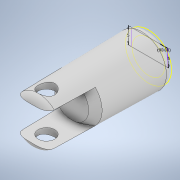
# Autodesk Inventor part: bicep
Saved by Autodesk Inventor 2021 (Build 250183000, 183)
## iProperties
Created: 2021-06-26
Part Number: bicep
Material: Generic
Document SubType Name: Modeling
Designer: TARUN
Density: 1 g/cm^3
Appearance: Default
Author: TARUN
Autodesk Inventor part; units mm, degrees
ref_plane "YZ Plane" through (0, 0, 0) normal (1, 0, 0) x (0, 1, 0)
ref_plane "XZ Plane" through (0, 0, 0) normal (0, 1, 0) x (-1, 0, 0)
ref_plane "XY Plane" through (0, 0, 0) normal (0, 0, 1) x (1, 0, 0)
sketch "Sketch1" plane through (0, 0, 0) normal (0, 0, 1) x (1, 0, 0)
  circle A0 centre (0, 0) radius 7.5
  dimension "d0" = 15
  constraints: 1 centre point, 1 coincident
  measures "d0" diameter of A0
extrude "Extrusion1" add sketch "Sketch1" along normal blind 35 draft -1
fillet "Fillet1" radius 2 2 edges at (-6.8891, 0, 35) (-7.5, 0, 0)
sketch "Sketch2" plane through (0, 0, 0) normal (0, 0, -1) x (-1, 0, 0)
  point P0 (0, 0)
sketch "Sketch3" plane through (0, 0, 0) normal (0, 0, -1) x (-1, 0, 0)
  circle A0 centre (0, 0) radius 4.9237 projected
  line L0 (0, 0) -> (5.0385, 0)
  line L1 (5.0385, 0) -> (5.0385, 5)
  line L2 (5.0385, 5) -> (-5.7641, 5)
  line L3 (-5.7641, 5) -> (-5.7641, 0)
  circle A1 centre (0, 0) radius 6.9234 projected
  line L4 (-5.7641, 0) -> (0, 0)
  dimension "d4" = 5
  dimension "d5" = 5
  dimension "d6" = 90
  constraints: 10 end point, 3 perpendicular, 1 horizontal
  measures "d4" distance of L0.end L1.end
  measures "d5" distance of L2.end L3.end
  measures "d6" angle of L3 L2
sketch "Sketch4" plane through (0, 0, 0) normal (0, 1, 0) x (-1, 0, 0)
  circle A0 centre (0, 30.571) radius 2.5
  point P0 (0, 0)
  dimension "d7" = 5
  constraints: 1 centre point
  measures "d7" diameter of A0
extrude "Extrusion2" cut sketch "Sketch4" against normal through all both and the other way through all
sketch "Sketch6" plane through (0, 0, 35) normal (0, 0, 1) x (1, 0, 0)
  arc A0 (-0.4232, 6.9104) -> (-0.4232, -6.9104) centre (0, 0) ccw projected
  line L0 (-4.7889, 5) -> (4.7889, 5)
  arc A1 (0.4232, -6.9104) -> (0.4232, 6.9104) centre (0, 0) ccw projected
  line L1 (-4.7889, 5) -> (-5.5424, 5)
  circle A2 centre (0, 0) radius 7.4645 projected
  line L2 (4.7889, 5) -> (5.5429, 5)
  line L3 (-5.5424, -5) -> (5.5424, -5)
  arc A3 (-5.5424, 5) -> (-5.5424, -5) centre (0, 0) ccw
  arc A4 (5.5424, -5) -> (5.5429, 5) centre (-0.0007, 0.0003) ccw
  point P0 (0, 0)
  dimension "d14" = 5
  dimension "d15" = 5
  constraints: 9 point on circle, 8 end point, 3 horizontal, 2 centre point, 1 concentric, 1 point on line
  measures "d14" distance from line of point (0, 0) L0
  measures "d15" distance from line of L3 point (0, 0)
extrude "Extrusion4" cut sketch "Sketch6" against normal blind 12 contours L0 A1 L3 A0 | A0 L3 A2 L1 | L2 A2 L3 A1
chamfer "Chamfer1" distance 2 angle 45 2 edges at (6.5634, -2.7038, 23) (-7.0985, 0, 23)
sketch "Sketch7" plane through (0, 0, 0) normal (0, 1, 0) x (-1, 0, 0)
  point P0 (0, 0)
body "Solid1"
